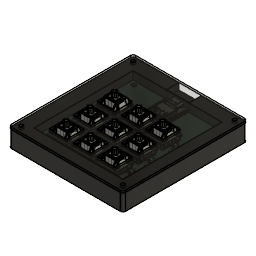
blandpad (Autodesk Fusion 360 archive; units mm, degrees)
design "Macro-final" references "Macro-final"
description: KiCad electronic assembly
part number: Macropad 1
description: Part Number
part number: UP_MX
part number: MX_UP
part number: MX_DOWN
part number: MX_PIN
part number: MX_CLICK
part number: D_DO-35_SOD27_P7.62mm_Horizontal
part number: Macropad_PCB
part number: Seeed Studio XIAO RP2040 v26
part number: MX_SPRING
Autodesk Fusion 360 part; units mm, degrees
sketch "Sketch1" plane through (0, 0, 0) normal (0, 0, 1) x (1, 0, 0)
  line L0 (-10.4, 35) -> (60, 35)
  line L1 (60, 35) -> (60, -43.4)
  line L2 (60, -43.4) -> (-10.4, -43.4)
  line L3 (-10.4, -43.4) -> (-10.4, 35)
  line L4 (-20.4, 45) -> (70, 45)
  line L5 (70, 45) -> (70, -53.4)
  line L6 (70, -53.4) -> (-20.4, -53.4)
  line L7 (-20.4, -53.4) -> (-20.4, 45)
  circle A0 centre (-15.4, 40) radius 1.45
  circle A1 centre (65, 40) radius 1.45
  circle A2 centre (65, -48.4) radius 1.45
  circle A3 centre (-15.4, -48.4) radius 1.45
  line L8 (-82.573, 9.1163) -> (-69.573, 9.1163)
  line L9 (-82.573, -4.8837) -> (-69.573, -4.8837)
  line L10 (-83.073, 8.6163) -> (-83.073, -4.3837)
  line L11 (-69.073, 8.6163) -> (-69.073, -4.3837)
  arc A4 (-82.573, 9.1163) -> (-83.073, 8.6163) centre (-82.573, 8.6163) ccw
  arc A5 (-69.073, 8.6163) -> (-69.573, 9.1163) centre (-69.573, 8.6163) ccw
  arc A6 (-83.073, -4.3837) -> (-82.573, -4.8837) centre (-82.573, -4.3837) ccw
  arc A7 (-69.573, -4.8837) -> (-69.073, -4.3837) centre (-69.573, -4.3837) ccw
  line L12 (-63.523, 9.1163) -> (-50.523, 9.1163)
  line L13 (-63.523, -4.8837) -> (-50.523, -4.8837)
  line L14 (-64.023, 8.6163) -> (-64.023, -4.3837)
  line L15 (-50.023, 8.6163) -> (-50.023, -4.3837)
  arc A8 (-63.523, 9.1163) -> (-64.023, 8.6163) centre (-63.523, 8.6163) ccw
  arc A9 (-50.023, 8.6163) -> (-50.523, 9.1163) centre (-50.523, 8.6163) ccw
  arc A10 (-64.023, -4.3837) -> (-63.523, -4.8837) centre (-63.523, -4.3837) ccw
  arc A11 (-50.523, -4.8837) -> (-50.023, -4.3837) centre (-50.523, -4.3837) ccw
  line L16 (-44.473, 9.1163) -> (-31.473, 9.1163)
  line L17 (-44.473, -4.8837) -> (-31.473, -4.8837)
  line L18 (-44.973, 8.6163) -> (-44.973, -4.3837)
  line L19 (-30.973, 8.6163) -> (-30.973, -4.3837)
  arc A12 (-44.473, 9.1163) -> (-44.973, 8.6163) centre (-44.473, 8.6163) ccw
  arc A13 (-30.973, 8.6163) -> (-31.473, 9.1163) centre (-31.473, 8.6163) ccw
  arc A14 (-44.973, -4.3837) -> (-44.473, -4.8837) centre (-44.473, -4.3837) ccw
  arc A15 (-31.473, -4.8837) -> (-30.973, -4.3837) centre (-31.473, -4.3837) ccw
  line L20 (-82.573, -9.9337) -> (-69.573, -9.9337)
  line L21 (-82.573, -23.9337) -> (-69.573, -23.9337)
  line L22 (-83.073, -10.4337) -> (-83.073, -23.4337)
  line L23 (-69.073, -10.4337) -> (-69.073, -23.4337)
  arc A16 (-82.573, -9.9337) -> (-83.073, -10.4337) centre (-82.573, -10.4337) ccw
  arc A17 (-69.073, -10.4337) -> (-69.573, -9.9337) centre (-69.573, -10.4337) ccw
  arc A18 (-83.073, -23.4337) -> (-82.573, -23.9337) centre (-82.573, -23.4337) ccw
  arc A19 (-69.573, -23.9337) -> (-69.073, -23.4337) centre (-69.573, -23.4337) ccw
  line L24 (-63.523, -9.9337) -> (-50.523, -9.9337)
  line L25 (-63.523, -23.9337) -> (-50.523, -23.9337)
  line L26 (-64.023, -10.4337) -> (-64.023, -23.4337)
  line L27 (-50.023, -10.4337) -> (-50.023, -23.4337)
  arc A20 (-63.523, -9.9337) -> (-64.023, -10.4337) centre (-63.523, -10.4337) ccw
  arc A21 (-50.023, -10.4337) -> (-50.523, -9.9337) centre (-50.523, -10.4337) ccw
  arc A22 (-64.023, -23.4337) -> (-63.523, -23.9337) centre (-63.523, -23.4337) ccw
  arc A23 (-50.523, -23.9337) -> (-50.023, -23.4337) centre (-50.523, -23.4337) ccw
  line L28 (-44.473, -9.9337) -> (-31.473, -9.9337)
  line L29 (-44.473, -23.9337) -> (-31.473, -23.9337)
  line L30 (-44.973, -10.4337) -> (-44.973, -23.4337)
  line L31 (-30.973, -10.4337) -> (-30.973, -23.4337)
  arc A24 (-44.473, -9.9337) -> (-44.973, -10.4337) centre (-44.473, -10.4337) ccw
  arc A25 (-30.973, -10.4337) -> (-31.473, -9.9337) centre (-31.473, -10.4337) ccw
  arc A26 (-44.973, -23.4337) -> (-44.473, -23.9337) centre (-44.473, -23.4337) ccw
  arc A27 (-31.473, -23.9337) -> (-30.973, -23.4337) centre (-31.473, -23.4337) ccw
  line L32 (-82.573, -28.9837) -> (-69.573, -28.9837)
  line L33 (-82.573, -42.9837) -> (-69.573, -42.9837)
  line L34 (-83.073, -29.4837) -> (-83.073, -42.4837)
  line L35 (-69.073, -29.4837) -> (-69.073, -42.4837)
  arc A28 (-82.573, -28.9837) -> (-83.073, -29.4837) centre (-82.573, -29.4837) ccw
  arc A29 (-69.073, -29.4837) -> (-69.573, -28.9837) centre (-69.573, -29.4837) ccw
  arc A30 (-83.073, -42.4837) -> (-82.573, -42.9837) centre (-82.573, -42.4837) ccw
  arc A31 (-69.573, -42.9837) -> (-69.073, -42.4837) centre (-69.573, -42.4837) ccw
  line L36 (-63.523, -28.9837) -> (-50.523, -28.9837)
  line L37 (-63.523, -42.9837) -> (-50.523, -42.9837)
  line L38 (-64.023, -29.4837) -> (-64.023, -42.4837)
  line L39 (-50.023, -29.4837) -> (-50.023, -42.4837)
  arc A32 (-63.523, -28.9837) -> (-64.023, -29.4837) centre (-63.523, -29.4837) ccw
  arc A33 (-50.023, -29.4837) -> (-50.523, -28.9837) centre (-50.523, -29.4837) ccw
  arc A34 (-64.023, -42.4837) -> (-63.523, -42.9837) centre (-63.523, -42.4837) ccw
  arc A35 (-50.523, -42.9837) -> (-50.023, -42.4837) centre (-50.523, -42.4837) ccw
  line L40 (-44.473, -28.9837) -> (-31.473, -28.9837)
  line L41 (-44.473, -42.9837) -> (-31.473, -42.9837)
  line L42 (-44.973, -29.4837) -> (-44.973, -42.4837)
  line L43 (-30.973, -29.4837) -> (-30.973, -42.4837)
  arc A36 (-44.473, -28.9837) -> (-44.973, -29.4837) centre (-44.473, -29.4837) ccw
  arc A37 (-30.973, -29.4837) -> (-31.473, -28.9837) centre (-31.473, -29.4837) ccw
  arc A38 (-44.973, -42.4837) -> (-44.473, -42.9837) centre (-44.473, -42.4837) ccw
  arc A39 (-31.473, -42.9837) -> (-30.973, -42.4837) centre (-31.473, -42.4837) ccw
  line L44 (-85.598, -45.5087) -> (-28.448, -45.5087)
  line L45 (-85.598, 11.6413) -> (-28.448, 11.6413)
  line L46 (-85.598, -45.5087) -> (-85.598, 11.6413)
  line L47 (-28.448, -45.5087) -> (-28.448, 11.6413)
  dimension "d1" = 70.4
  dimension "d2" = 78.4
  dimension "d3" = 10
  dimension "d4" = 10
  dimension "d5" = 10
  dimension "d6" = 10
  dimension "d7" = 2.9
  dimension "d8" = 5
  dimension "d10" = 2.9
  dimension "d11" = 2.9
  dimension "d12" = 5
  dimension "d13" = 5
  dimension "d14" = 2.9
  dimension "d15" = 5
  dimension "d16" = 5
  constraint horizontal L0
  constraint vertical L1
  constraint horizontal L2
  constraint vertical L3
  constraint horizontal L4
  constraint vertical L5
  constraint horizontal L6
  constraint vertical L7
  measures "d1" distance of L1 L3
  measures "d2" distance of L0 L2
  measures "d3" distance of L0 L4
  measures "d4" distance of L2 L6
  measures "d5" distance of L1 L5
  measures "d6" distance of L3 L7
  measures "d7" diameter of A0
  measures "d8" distance of L7 A0.centre
  measures "d10" diameter of A1
  measures "d11" diameter of A2
  measures "d12" distance of L6 A2.centre
  measures "d13" distance of L5 A2.centre
  measures "d14" diameter of A3
  measures "d15" distance of L7 A3.centre
  measures "d16" distance of L6 A3.centre
extrude "Extrude1" add sketch "Sketch1" along normal blind 13 contours L4 L5 L6 L7 makes body 1
extrude "Extrude2" add sketch "Sketch1" along normal blind 3 contours L0 L1 L2 L3 bodies 1
move_body "Move1" bodies 1 to x (1, 0, 0) y (0, 1, 0) z (0, 0, 1) at (-20.5263, 4.3029, -4.6889)
sketch "plate-2026-03-23T10_31_19.720Z" plane through (0, 0, 0) normal (0, 0, 1) x (1, 0, 0)
  line L0 (-22.3071, 26.2615) -> (-9.3071, 26.2615)
  line L1 (-22.3071, 12.2615) -> (-9.3071, 12.2615)
  line L2 (-22.8071, 25.7615) -> (-22.8071, 12.7615)
  line L3 (-8.8071, 25.7615) -> (-8.8071, 12.7615)
  arc A0 (-22.3071, 26.2615) -> (-22.8071, 25.7615) centre (-22.3071, 25.7615) ccw
  arc A1 (-8.8071, 25.7615) -> (-9.3071, 26.2615) centre (-9.3071, 25.7615) ccw
  arc A2 (-22.8071, 12.7615) -> (-22.3071, 12.2615) centre (-22.3071, 12.7615) ccw
  arc A3 (-9.3071, 12.2615) -> (-8.8071, 12.7615) centre (-9.3071, 12.7615) ccw
  line L4 (-3.2571, 26.2615) -> (9.7429, 26.2615)
  line L5 (-3.2571, 12.2615) -> (9.7429, 12.2615)
  line L6 (-3.7571, 25.7615) -> (-3.7571, 12.7615)
  line L7 (10.2429, 25.7615) -> (10.2429, 12.7615)
  arc A4 (-3.2571, 26.2615) -> (-3.7571, 25.7615) centre (-3.2571, 25.7615) ccw
  arc A5 (10.2429, 25.7615) -> (9.7429, 26.2615) centre (9.7429, 25.7615) ccw
  arc A6 (-3.7571, 12.7615) -> (-3.2571, 12.2615) centre (-3.2571, 12.7615) ccw
  arc A7 (9.7429, 12.2615) -> (10.2429, 12.7615) centre (9.7429, 12.7615) ccw
  line L8 (15.7929, 26.2615) -> (28.7929, 26.2615)
  line L9 (15.7929, 12.2615) -> (28.7929, 12.2615)
  line L10 (15.2929, 25.7615) -> (15.2929, 12.7615)
  line L11 (29.2929, 25.7615) -> (29.2929, 12.7615)
  arc A8 (15.7929, 26.2615) -> (15.2929, 25.7615) centre (15.7929, 25.7615) ccw
  arc A9 (29.2929, 25.7615) -> (28.7929, 26.2615) centre (28.7929, 25.7615) ccw
  arc A10 (15.2929, 12.7615) -> (15.7929, 12.2615) centre (15.7929, 12.7615) ccw
  arc A11 (28.7929, 12.2615) -> (29.2929, 12.7615) centre (28.7929, 12.7615) ccw
  line L12 (-22.3071, 7.2115) -> (-9.3071, 7.2115)
  line L13 (-22.3071, -6.7885) -> (-9.3071, -6.7885)
  line L14 (-22.8071, 6.7115) -> (-22.8071, -6.2885)
  line L15 (-8.8071, 6.7115) -> (-8.8071, -6.2885)
  arc A12 (-22.3071, 7.2115) -> (-22.8071, 6.7115) centre (-22.3071, 6.7115) ccw
  arc A13 (-8.8071, 6.7115) -> (-9.3071, 7.2115) centre (-9.3071, 6.7115) ccw
  arc A14 (-22.8071, -6.2885) -> (-22.3071, -6.7885) centre (-22.3071, -6.2885) ccw
  arc A15 (-9.3071, -6.7885) -> (-8.8071, -6.2885) centre (-9.3071, -6.2885) ccw
  line L16 (-3.2571, 7.2115) -> (9.7429, 7.2115)
  line L17 (-3.2571, -6.7885) -> (9.7429, -6.7885)
  line L18 (-3.7571, 6.7115) -> (-3.7571, -6.2885)
  line L19 (10.2429, 6.7115) -> (10.2429, -6.2885)
  arc A16 (-3.2571, 7.2115) -> (-3.7571, 6.7115) centre (-3.2571, 6.7115) ccw
  arc A17 (10.2429, 6.7115) -> (9.7429, 7.2115) centre (9.7429, 6.7115) ccw
  arc A18 (-3.7571, -6.2885) -> (-3.2571, -6.7885) centre (-3.2571, -6.2885) ccw
  arc A19 (9.7429, -6.7885) -> (10.2429, -6.2885) centre (9.7429, -6.2885) ccw
  line L20 (15.7929, 7.2115) -> (28.7929, 7.2115)
  line L21 (15.7929, -6.7885) -> (28.7929, -6.7885)
  line L22 (15.2929, 6.7115) -> (15.2929, -6.2885)
  line L23 (29.2929, 6.7115) -> (29.2929, -6.2885)
  arc A20 (15.7929, 7.2115) -> (15.2929, 6.7115) centre (15.7929, 6.7115) ccw
  arc A21 (29.2929, 6.7115) -> (28.7929, 7.2115) centre (28.7929, 6.7115) ccw
  arc A22 (15.2929, -6.2885) -> (15.7929, -6.7885) centre (15.7929, -6.2885) ccw
  arc A23 (28.7929, -6.7885) -> (29.2929, -6.2885) centre (28.7929, -6.2885) ccw
  line L24 (-22.3071, -11.8385) -> (-9.3071, -11.8385)
  line L25 (-22.3071, -25.8385) -> (-9.3071, -25.8385)
  line L26 (-22.8071, -12.3385) -> (-22.8071, -25.3385)
  line L27 (-8.8071, -12.3385) -> (-8.8071, -25.3385)
  arc A24 (-22.3071, -11.8385) -> (-22.8071, -12.3385) centre (-22.3071, -12.3385) ccw
  arc A25 (-8.8071, -12.3385) -> (-9.3071, -11.8385) centre (-9.3071, -12.3385) ccw
  arc A26 (-22.8071, -25.3385) -> (-22.3071, -25.8385) centre (-22.3071, -25.3385) ccw
  arc A27 (-9.3071, -25.8385) -> (-8.8071, -25.3385) centre (-9.3071, -25.3385) ccw
  line L28 (-3.2571, -11.8385) -> (9.7429, -11.8385)
  line L29 (-3.2571, -25.8385) -> (9.7429, -25.8385)
  line L30 (-3.7571, -12.3385) -> (-3.7571, -25.3385)
  line L31 (10.2429, -12.3385) -> (10.2429, -25.3385)
  arc A28 (-3.2571, -11.8385) -> (-3.7571, -12.3385) centre (-3.2571, -12.3385) ccw
  arc A29 (10.2429, -12.3385) -> (9.7429, -11.8385) centre (9.7429, -12.3385) ccw
  arc A30 (-3.7571, -25.3385) -> (-3.2571, -25.8385) centre (-3.2571, -25.3385) ccw
  arc A31 (9.7429, -25.8385) -> (10.2429, -25.3385) centre (9.7429, -25.3385) ccw
  line L32 (15.7929, -11.8385) -> (28.7929, -11.8385)
  line L33 (15.7929, -25.8385) -> (28.7929, -25.8385)
  line L34 (15.2929, -12.3385) -> (15.2929, -25.3385)
  line L35 (29.2929, -12.3385) -> (29.2929, -25.3385)
  arc A32 (15.7929, -11.8385) -> (15.2929, -12.3385) centre (15.7929, -12.3385) ccw
  arc A33 (29.2929, -12.3385) -> (28.7929, -11.8385) centre (28.7929, -12.3385) ccw
  arc A34 (15.2929, -25.3385) -> (15.7929, -25.8385) centre (15.7929, -25.3385) ccw
  arc A35 (28.7929, -25.8385) -> (29.2929, -25.3385) centre (28.7929, -25.3385) ccw
  line L36 (-25.3321, -28.3635) -> (31.8179, -28.3635)
  line L37 (-25.3321, 28.7865) -> (31.8179, 28.7865)
  line L38 (-25.3321, -28.3635) -> (-25.3321, 28.7865)
  line L39 (31.8179, -28.3635) -> (31.8179, 28.7865)
extrude "Extrude3" add sketch "plate-2026-03-23T10_31_19.720Z" along normal blind 3 separate body makes body 2
